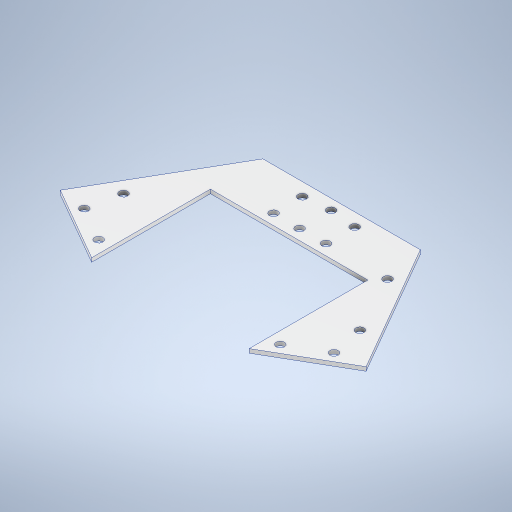
# Autodesk Inventor part: flame_upper_back
Saved by Autodesk Inventor 2024.1 (Build 281209000, 209)
## iProperties
Created: 2025-03-06
Part Number: flame_upper_back
Material: アルミニウム 6061
Document SubType Name: Sheet Metal
Designer: hibik
Density: 2.7 g/cm^3
Sheet Metal Rule: Default_mm
Appearance: アルミニウム - フラット
Author: hibik
Autodesk Inventor part; units mm, degrees
ref_plane "YZ Plane" through (0, 0, 0) normal (1, 0, 0) x (0, 1, 0)
ref_plane "XZ Plane" through (0, 0, 0) normal (0, 1, 0) x (-1, 0, 0)
ref_plane "XY Plane" through (0, 0, 0) normal (0, 0, 1) x (1, 0, 0)
sketch "スケッチ1" plane through (0, 0, 0) normal (0, 1, 0) x (-1, 0, 0)
  line L0 (0, 0) -> (-30, 0)
  line L1 (-30, 0) -> (-58.25, 48.9304)
  line L2 (-58.25, 48.9304) -> (-30, 65.2406)
  line L3 (-30, 65.2406) -> (0, 65.2406)
  line L4 (0, 65.2406) -> (0, 0)
  line L5 (0, 0) -> (30, 0)
  line L6 (30, 0) -> (58.25, 48.9304)
  line L7 (58.25, 48.9304) -> (30, 65.2406)
  line L8 (30, 65.2406) -> (0, 65.2406)
  line L9 (-30, 65.2406) -> (-30, 20)
  line L10 (-30, 20) -> (30, 20)
  line L11 (30, 20) -> (30, 65.2406)
  dimension "d0" = 60
  dimension "d1" = 30
  dimension "d3" = 56.5
  dimension "d4" = 20
  measures "d0" angle of L0 L1
  measures "d1" distance of L0.start L0.end
  measures "d3" distance from line of L0.end L2
  measures "d4" distance between parallel lines of L5 L10
extrude "プレート1" add sketch "スケッチ1" along normal blind 1.5 contours L0 L1 L2 L9 L10 L4 | L4 L10 L11 L7 L6 L5
sketch "スケッチ2" plane through (0, 1.5, 0) normal (0, 1, 0) x (1, 0, 0)
  circle A0 centre (33.4199, -15.9234) radius 1.35 projected
  circle A1 centre (10, -5) radius 1.35 projected
  circle A2 centre (45.0538, -38.074) radius 1.35 projected
  line L0 (30, 0) -> (5, 0) projected
  line L1 (5, 0) -> (5, -20) projected
  line L2 (5, -20) -> (24.2265, -20) projected
  line L3 (24.2265, -20) -> (39.7596, -46.9042) projected
  line L4 (39.7596, -46.9042) -> (52.75, -39.4042) projected
  line L5 (52.75, -39.4042) -> (30, 0) projected
  circle A3 centre (-45.0538, -38.074) radius 1.35 projected
  circle A4 centre (-25.5276, -26.2535) radius 1.35 projected
  circle A5 centre (-10, -5) radius 1.35 projected
  line L6 (-42.0628, -34.8934) -> (-47.259, -31.8934) projected
  line L7 (-47.259, -31.8934) -> (-51.884, -39.9042) projected
  line L8 (-51.884, -39.9042) -> (-33.6974, -50.4042) projected
  line L9 (-33.6974, -50.4042) -> (-16.1436, -20) projected
  line L10 (-16.1436, -20) -> (-5, -20) projected
  line L11 (-5, -20) -> (-5, 0) projected
  line L12 (-5, 0) -> (-30, 0) projected
  line L13 (-30, 0) -> (-29.134, -0.5) projected
  line L14 (-29.134, -0.5) -> (-33.759, -8.5107) projected
  line L15 (-33.759, -8.5107) -> (-28.5628, -11.5107) projected
  line L16 (-28.5628, -11.5107) -> (-31.5628, -16.7069) projected
  line L17 (-31.5628, -16.7069) -> (-36.759, -13.7069) projected
  line L18 (-36.759, -13.7069) -> (-44.259, -26.6973) projected
  line L19 (-44.259, -26.6973) -> (-39.0628, -29.6973) projected
  line L20 (-39.0628, -29.6973) -> (-42.0628, -34.8934) projected
  circle A6 centre (10, -15.9234) radius 1.6
  circle A7 centre (-10, -15.9234) radius 1.6
  circle A8 centre (45.0538, -38.074) radius 1.6
  circle A9 centre (33.4199, -15.9234) radius 1.6
  circle A10 centre (10, -5) radius 1.6
  circle A11 centre (-10, -5) radius 1.6
  circle A12 centre (-45.0538, -38.074) radius 1.6
  point P0 (0, 0)
  dimension "d15" = 3.2
  constraints: 7 centre point, 6 equal radius, 5 coincident, 2 horizontal alignment, 2 vertical alignment
  measures "d15" diameter of A6
extrude "切り取り1" cut sketch "スケッチ2" against normal blind 1.5 contours A0 | A1 | A2 | A3 | A5 | A6 | A7 | A8 | A9 | A10 | A11 | A12
sketch "スケッチ3" plane through (0, 1.5, 0) normal (0, 1, 0) x (1, 0, 0)
  circle A0 centre (-34.5994, -57.9663) radius 1.35 projected
  circle A1 centre (-47.5897, -50.4663) radius 1.35 projected
  circle A2 centre (-34.5994, -57.9663) radius 1.6
  circle A3 centre (-47.5897, -50.4663) radius 1.6
  line L0 (0, 0) -> (0, -17.1594)
  circle A4 centre (34.5994, -57.9663) radius 1.6
  circle A5 centre (47.5897, -50.4663) radius 1.6
  dimension "d7" = 3.2
  dimension "d8" = 3.2
  constraints: 4 centre point, 2 coincident, 2 end point, 2 symmetric about line, 1 vertical, 2 other
  measures "d7" diameter of A2
  measures "d8" diameter of A3
extrude "切り取り2" cut sketch "スケッチ3" against normal blind 1.5 contours A0 | A1 | A2 | A3 | A4 | A5
sketch "スケッチ4" plane through (0, 1.5, 0) normal (0, 1, 0) x (1, 0, 0)
  line L0 (5, 0) -> (5, -20) projected
  line L1 (-5, -20) -> (-5, 0) projected
  circle A0 centre (0, -16) radius 1.6
  circle A1 centre (0, -4) radius 1.6
  line L2 (5, -10) -> (-5, -10)
  line L3 (-30, 0) -> (30, 0) projected
  point P0 (0, 0)
  point P1 (0, 0)
  point P2 (0, 0)
  dimension "d11" = 3.2
  dimension "d12" = 12
  constraints: 4 midpoint, 2 centre point, 2 end point, 2 vertical alignment, 1 equal radius, 1 symmetric about line
  measures "d11" diameter of A0
  measures "d12" distance of A1.centre A0.centre
extrude "切り取り3" cut sketch "スケッチ4" against normal blind 1.5 contours A0 | A1
equation "\"d5\" = Thickness"
equation "\"d9\" = Thickness"
equation "\"d13\" = Thickness"
equation "\"d2\" = Thickness"
equation "\"BendRadius\" = Thickness"
equation "\"BendReliefWidth\" = Thickness"
equation "\"BendReliefDepth\" = 0.5 * Thickness"
equation "\"CornerReliefSize\" = 4 * Thickness"
equation "\"MinimumRemnant\" = 2 * Thickness"
equation "\"TransitionRadius\" = BendRadius"
equation "\"JacobiRadiusSize\" = BendRadius"
equation "\"GapSize\" = Thickness"
equation "\"Thickness\" = 1.5"
